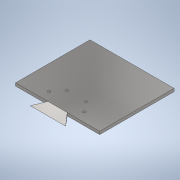
# Autodesk Inventor part: Part12
Saved by Autodesk Inventor 2022.3 (Build 263350000, 350)
## iProperties
Created: 2022-11-17
Part Number: Part12
Material: Steel, Alloy
Document SubType Name: Modeling
Designer: komputer
Density: 7.73 g/cm^3
Appearance: Semi-Polished
Mass: 236.899 g
Surface Area: 193.708 cm^2
Volume: 30.6467 cm^3
Author: komputer
Autodesk Inventor part; units mm, degrees
ref_plane "YZ Plane" through (0, 0, 0) normal (1, 0, 0) x (0, 1, 0)
ref_plane "XZ Plane" through (0, 0, 0) normal (0, 1, 0) x (-1, 0, 0)
ref_plane "XY Plane" through (0, 0, 0) normal (0, 0, 1) x (1, 0, 0)
sketch "Sketch1" plane through (0, 0, 0) normal (0, 1, 0) x (-1, 0, 0)
  line L0 (-8.4349, 11.6133) -> (91.5651, 11.6133)
  line L1 (91.5651, 11.6133) -> (91.5651, -88.3867)
  line L2 (91.5651, -88.3867) -> (-8.4349, -88.3867)
  line L3 (-8.4349, -88.3867) -> (-8.4349, 11.6133)
  point P0 (0, 0)
  dimension "d0" = 100
  dimension "d1" = 100
  constraints: 8 end point, 2 parallel, 1 horizontal, 1 perpendicular
  measures "d0" distance of L1.end L2.end
  measures "d1" distance of L0.end L1.end
extrude "Extrusion1" add sketch "Sketch1" along normal blind 3.5
sketch "Sketch2" plane through (-91.5651, 0, -88.3867) normal (-1, 0, 0) x (0, 0, 1)
  line L0 (0, 0) -> (100, 0) projected
  line L1 (100, 0) -> (100, 3.5) projected
  line L2 (0, 3.5) -> (100, 3.5) projected
  line L3 (0, 0) -> (0, 3.5) projected
  line L4 (0, 3.5) -> (100, 3.5) projected
  line L5 (100, 3.5) -> (90, 3.5)
  line L6 (0, 0) -> (100, 0) projected
  line L7 (90, 3.5) -> (100, 0)
  point P0 (88.3867, 0)
  dimension "d4" = 10
  constraints: 4 end point, 1 point on line
  measures "d4" distance of L1.end L5.end
extrude "Extrusion2" cut sketch "Sketch2" against normal through all contours L7 L2 L1
sketch "Sketch3" plane through (0, 3.5, 0) normal (0, 1, 0) x (1, 0, 0)
  line L0 (-91.5651, -1.6133) -> (8.4349, -1.6133) projected
  line L1 (8.4349, -1.6133) -> (8.4349, 88.3867) projected
  line L2 (8.4349, 88.3867) -> (-91.5651, 88.3867) projected
  line L3 (-91.5651, 88.3867) -> (-91.5651, -1.6133) projected
  line L4 (8.4349, -1.6133) -> (8.4349, -11.6133) projected
  line L5 (-91.5651, -1.6133) -> (8.4349, -1.6133) projected
  line L6 (-91.5651, -11.6133) -> (-91.5651, -1.6133) projected
  line L7 (-91.5651, -11.6133) -> (8.4349, -11.6133) projected
  line L8 (-91.5651, -11.6133) -> (8.4349, -11.6133) projected
  line L9 (8.4349, 88.3867) -> (-91.5651, 88.3867) projected
  line L10 (-91.5651, 88.3867) -> (-91.5651, -11.6133) projected
  line L11 (-41.5651, -11.6133) -> (8.4349, -11.6133)
  line L12 (-91.5651, -11.6133) -> (-41.5651, -11.6133)
  line L13 (-16.5651, -11.6133) -> (8.4349, -11.6133)
  line L14 (-91.5651, -11.6133) -> (-66.5651, -11.6133)
  line L15 (-16.5651, -11.6133) -> (-4.0651, -11.6133)
  line L16 (-79.0651, -11.6133) -> (-66.5651, -11.6133)
  line L17 (-41.5651, 25.8867) -> (-72.8151, -11.6133)
  line L18 (-41.5651, 25.8867) -> (-10.3151, -11.6133)
  line L19 (-28.2288, 9.8831) -> (-18.6484, -1.6133)
  line L20 (-91.5651, -1.6133) -> (8.4349, -1.6133) projected
  circle A0 centre (-30.1493, 12.1878) radius 1.6
  circle A1 centre (-20.569, 0.6914) radius 1.6
  line L21 (-18.6484, -1.6133) -> (-20.569, 0.6914)
  line L22 (-41.5651, 25.8867) -> (-41.5651, -11.6133)
  circle A2 centre (-52.9808, 12.1878) radius 1.6
  circle A3 centre (-62.5612, 0.6914) radius 1.6
  point P0 (0, 0)
  point P1 (-63.1373, 0)
  dimension "d15" = 3.2
  dimension "d16" = 3.2
  dimension "d17" = 3
  constraints: 22 end point, 7 midpoint, 6 point on line, 5 collinear, 4 centre point, 2 horizontal, 2 symmetric about line, 1 vertical, 2 other
  measures "d15" diameter of A0
  measures "d16" diameter of A1
  measures "d17" distance of L21.start L21.end
extrude "Extrusion3" cut sketch "Sketch3" against normal through all contours A1 L18 | L18 A1 | A3 L17 | L17 A3 | A2 L17 | L17 A2 | A0 L18 | L18 A0
sketch "Sketch4" plane through (0, 0, 0) normal (0, -1, 0) x (1, 0, 0)
  circle A0 centre (-52.9808, -12.1878) radius 1.6 projected
  circle A1 centre (-20.569, -0.6914) radius 1.6 projected
  circle A2 centre (-62.5612, -0.6914) radius 1.6 projected
  circle A3 centre (-30.1493, -12.1878) radius 1.6 projected
  line L0 (8.4349, -88.3867) -> (-91.5651, -88.3867) projected
  line L1 (8.4349, 11.6133) -> (8.4349, -88.3867) projected
  line L2 (-91.5651, 11.6133) -> (8.4349, 11.6133) projected
  line L3 (-91.5651, -88.3867) -> (-91.5651, 11.6133) projected
  line L4 (-91.5651, -88.3867) -> (-91.5651, 11.6133) projected
  line L5 (-91.5651, 11.6133) -> (8.4349, 11.6133)
  line L6 (8.4349, 11.6133) -> (8.4349, 21.6133)
  line L7 (8.4349, 21.6133) -> (-91.5651, 21.6133)
  line L8 (-91.5651, 21.6133) -> (-91.5651, 11.6133)
  line L9 (8.4349, 11.6133) -> (8.4349, -88.3867) projected
  line L10 (-91.5651, -88.3867) -> (8.4349, -88.3867)
  line L11 (8.4349, -88.3867) -> (8.4349, -78.3867)
  line L12 (8.4349, -78.3867) -> (-91.5651, -78.3867)
  line L13 (-91.5651, -78.3867) -> (-91.5651, -88.3867)
  line L14 (-91.5651, 1.6133) -> (8.4349, 1.6133) projected
  line L15 (-91.5651, 11.6133) -> (8.4349, 11.6133)
  line L16 (8.4349, 11.6133) -> (8.4349, 1.6133)
  line L17 (8.4349, 1.6133) -> (-91.5651, 1.6133)
  line L18 (-91.5651, 1.6133) -> (-91.5651, 11.6133)
  ellipse E0 centre (-76.8987, 15.9252) end of major axis (-87.6538, 6.9626) minor radius 2.0831 projected
  point P0 (0, 0)
  dimension "d20" = 10
  dimension "d21" = 10
  constraints: 24 end point, 6 parallel, 3 horizontal, 3 perpendicular, 1 point on line, 1 other
  measures "d20" distance of L6.end L5.end
  measures "d21" distance of L11.end L10.end
extrude "Extrusion4" add sketch "Sketch4" against normal up to surface (3.5 mm away) contours L14 L3 L2 E0 L1 | L2 E0 L7 L6 | L8 L7 E0 L2 | E0 L2 | L2 E0 L7
sketch "Sketch5" plane through (0, 0, 0) normal (0, -1, 0) x (1, 0, 0)
  line L0 (-91.5651, -88.3867) -> (-91.5651, 21.6133) projected
  line L1 (8.4349, -88.3867) -> (-91.5651, -88.3867) projected
  line L2 (8.4349, -88.3867) -> (8.4349, 21.6133) projected
  line L3 (8.4349, 21.6133) -> (-91.5651, 21.6133) projected
  circle A0 centre (-30.1493, -12.1878) radius 1.6 projected
  circle A1 centre (-62.5612, -0.6914) radius 1.6 projected
  circle A2 centre (-20.569, -0.6914) radius 1.6 projected
  circle A3 centre (-52.9808, -12.1878) radius 1.6 projected
  line L4 (-91.5651, -88.3867) -> (-91.5651, 21.6133) projected
  line L5 (8.4349, -88.3867) -> (-91.5651, -88.3867)
  line L6 (-91.5651, -88.3867) -> (-91.5651, -78.3867)
  line L7 (-91.5651, -78.3867) -> (8.4349, -78.3867)
  line L8 (8.4349, -78.3867) -> (8.4349, -88.3867)
  point P0 (0, 0)
  dimension "d24" = 10
  constraints: 8 end point, 2 parallel, 1 horizontal, 1 perpendicular, 1 point on line
  measures "d24" distance of L5.end L6.end
extrude "Extrusion5" cut sketch "Sketch5" against normal through all contours L0 L7 L2 L1
sketch "Sketch6" plane through (-91.5651, 0, 21.6133) normal (-1, 0, 0) x (0, 0, 1)
  line L0 (-100, 3.5) -> (-100, 0) projected
  line L1 (-100, 0) -> (0, 0) projected
  line L2 (0, 0) -> (0, 3.5) projected
  line L3 (0, 3.5) -> (-100, 3.5) projected
  line L4 (-6.5312, 3.5) -> (-20.2018, 3.5) projected
  line L5 (-6.5312, 8.5) -> (-6.5312, 3.5) projected
  line L6 (-20.2018, 8.5) -> (-6.5312, 8.5) projected
  line L7 (-20.2018, 3.5) -> (-20.2018, 8.5) projected
  line L8 (-100, 0) -> (0, 0) projected
  line L9 (0, 0) -> (-11.4782, 3.5)
  line L10 (0, 3.5) -> (-100, 3.5) projected
  point P0 (-21.6133, 0)
  dimension "d27" = 12
  constraints: 2 end point, 1 point on line
  measures "d27" distance of L1.end L9.end
extrude "Extrusion6" cut sketch "Sketch6" against normal through all contours L9 L3 L2
sketch "Sketch7" plane through (0, 3.5, 0) normal (0, 1, 0) x (1, 0, 0)
  line L0 (-91.5651, -10.1351) -> (8.4349, -10.1351) projected
  line L1 (8.4349, -10.1351) -> (8.4349, 78.3867) projected
  line L2 (8.4349, 78.3867) -> (-91.5651, 78.3867) projected
  line L3 (-91.5651, -10.1351) -> (-91.5651, 78.3867) projected
  circle A0 centre (-52.9808, 12.1878) radius 1.6 projected
  circle A1 centre (-20.569, 0.6914) radius 1.6 projected
  circle A2 centre (-62.5612, 0.6914) radius 1.6 projected
  circle A3 centre (-30.1493, 12.1878) radius 1.6 projected
  line L4 (8.4349, -10.1351) -> (8.4349, -21.6133) projected
  line L5 (-91.5651, -10.1351) -> (8.4349, -10.1351) projected
  line L6 (-91.5651, -21.6133) -> (-91.5651, -10.1351) projected
  line L7 (8.4349, -21.6133) -> (-91.5651, -21.6133) projected
  circle A4 centre (-30.1493, 12.1878) radius 1.6 projected
  circle A5 centre (-20.569, 0.6914) radius 1.6 projected
  line L8 (-30.1493, 12.1878) -> (-20.569, 0.6914)
  line L9 (-91.5651, -10.1351) -> (8.4349, -10.1351) projected
  line L10 (-30.1493, -10.1351) -> (-20.569, -21.6133)
  line L11 (8.4349, -21.6133) -> (-91.5651, -21.6133) projected
  circle A6 centre (-62.5612, 0.6914) radius 1.6 projected
  line L12 (-52.9808, 12.1878) -> (-62.5612, 0.6914)
  line L13 (-52.9808, -10.1351) -> (-62.5612, -21.6133)
  point P0 (0, 0)
  constraints: 8 end point, 4 point on line
extrude "Extrusion7" cut sketch "Sketch7" against normal blind 10 contours L0 L13 L7 L6 | L0 L4 L7 L10
sketch "Sketch8" plane through (0, 3.5, 0) normal (0, 1, 0) x (1, 0, 0)
  line L0 (-91.5651, -10.1351) -> (-52.9808, -10.1351) projected
  line L1 (-52.9808, -10.1351) -> (-30.1493, -10.1351) projected
  line L2 (-30.1493, -10.1351) -> (8.4349, -10.1351) projected
  line L3 (8.4349, -10.1351) -> (8.4349, 78.3867) projected
  line L4 (8.4349, 78.3867) -> (-91.5651, 78.3867) projected
  line L5 (-91.5651, -10.1351) -> (-91.5651, 78.3867) projected
  circle A0 centre (-52.9808, 12.1878) radius 1.6 projected
  circle A1 centre (-20.569, 0.6914) radius 1.6 projected
  circle A2 centre (-62.5612, 0.6914) radius 1.6 projected
  circle A3 centre (-30.1493, 12.1878) radius 1.6 projected
  line L6 (8.4349, -10.1351) -> (8.4349, 78.3867) projected
  line L7 (8.4349, -10.1351) -> (-30.1493, -10.1351)
  line L8 (-30.1493, -10.1351) -> (-30.1493, -7.1351)
  line L9 (-30.1493, -7.1351) -> (8.4349, -7.1351)
  line L10 (8.4349, -7.1351) -> (8.4349, -10.1351)
  line L11 (-91.5651, -10.1351) -> (-52.9808, -10.1351)
  line L12 (-52.9808, -10.1351) -> (-52.9808, -7.1351)
  line L13 (-52.9808, -7.1351) -> (-91.5651, -7.1351)
  line L14 (-91.5651, -7.1351) -> (-91.5651, -10.1351)
  point P0 (0, 0)
  dimension "d32" = 3
  constraints: 16 end point, 4 parallel, 2 horizontal, 2 perpendicular, 1 point on line
  measures "d32" distance of L7.end L8.end
extrude "Extrusion8" cut sketch "Sketch8" against normal through all contours L5 L13 L12 L0 | L8 L9 L3 L2
sketch "Sketch9" plane through (0, 3.5, 0) normal (0, 1, 0) x (1, 0, 0)
  circle A0 centre (-30.1493, 12.1878) radius 1.6 projected
  circle A1 centre (-62.5612, 0.6914) radius 1.6 projected
  circle A2 centre (-20.569, 0.6914) radius 1.6 projected
  circle A3 centre (-52.9808, 12.1878) radius 1.6 projected
  line L0 (-91.5651, -7.1351) -> (-52.9808, -7.1351) projected
  line L1 (-52.9808, -7.1351) -> (-52.9808, -10.1351) projected
  line L2 (-52.9808, -10.1351) -> (-30.1493, -10.1351) projected
  line L3 (-30.1493, -10.1351) -> (-30.1493, -7.1351) projected
  line L4 (-30.1493, -7.1351) -> (8.4349, -7.1351) projected
  line L5 (8.4349, -7.1351) -> (8.4349, 78.3867) projected
  line L6 (8.4349, 78.3867) -> (-91.5651, 78.3867) projected
  line L7 (-91.5651, -7.1351) -> (-91.5651, 78.3867) projected
  line L8 (-91.5651, 78.3867) -> (-91.5651, -7.1351) projected
  line L9 (8.4349, 78.3867) -> (8.4349, -7.1351) projected
  line L10 (-91.5651, 78.3867) -> (8.4349, 78.3867)
  line L11 (8.4349, 78.3867) -> (8.4349, 73.3867)
  line L12 (8.4349, 73.3867) -> (-91.5651, 73.3867)
  line L13 (-91.5651, 73.3867) -> (-91.5651, 78.3867)
  line L14 (-91.5651, 78.3867) -> (8.4349, 78.3867) projected
  line L15 (-41.5651, 78.3867) -> (-41.5651, 59.9995)
  line L16 (-41.5651, 59.9995) -> (-16.5651, 59.9995)
  line L17 (-16.5651, 59.9995) -> (-66.5651, 59.9995)
  line L18 (8.4349, 73.3867) -> (-16.5651, 73.3867)
  line L19 (-16.5651, 73.3867) -> (-16.5651, 45.3867)
  line L20 (-16.5651, 45.3867) -> (8.4349, 45.3867)
  line L21 (8.4349, 45.3867) -> (8.4349, 73.3867)
  line L22 (-66.5651, 73.3867) -> (-79.5403, 73.3867)
  line L23 (-79.5403, 73.3867) -> (-79.5403, 45.3867)
  line L24 (-79.5403, 45.3867) -> (-66.5651, 45.3867)
  line L25 (-66.5651, 45.3867) -> (-66.5651, 73.3867)
  line L26 (-91.5651, 45.3867) -> (-66.5651, 45.3867)
  line L27 (-66.5651, 45.3867) -> (-66.5651, 78.3867)
  line L28 (-66.5651, 78.3867) -> (-91.5651, 78.3867)
  line L29 (-91.5651, 78.3867) -> (-91.5651, 45.3867)
  line L30 (-14.4969, 45.3867) -> (-14.4969, 50.3867)
  line L31 (-14.4969, 50.3867) -> (-14.4969, 78.3867)
  line L32 (-14.4969, 64.3867) -> (-82.4701, 64.3867)
  line L33 (-82.4701, 64.3867) -> (-3.1512, 64.3867)
  line L34 (-14.4969, 64.3867) -> (-9.1279, 64.3867)
  line L35 (-9.1279, 64.3867) -> (-9.1279, 62.3867)
  line L36 (-9.1279, 62.3867) -> (-14.4969, 62.3867)
  line L37 (-14.4969, 62.3867) -> (-14.4969, 64.3867)
  line L38 (-14.4969, 64.3867) -> (-9.1279, 64.3867)
  line L39 (-9.1279, 64.3867) -> (-9.1279, 66.3867)
  line L40 (-9.1279, 66.3867) -> (-14.4969, 66.3867)
  line L41 (-14.4969, 66.3867) -> (-14.4969, 64.3867)
  line L42 (-66.5651, 64.3867) -> (-72.2729, 64.3867)
  line L43 (-72.2729, 64.3867) -> (-72.2729, 62.3867)
  line L44 (-72.2729, 62.3867) -> (-66.5651, 62.3867)
  line L45 (-66.5651, 62.3867) -> (-66.5651, 64.3867)
  line L46 (-72.2729, 62.3867) -> (-66.5651, 62.3867)
  line L47 (-66.5651, 62.3867) -> (-66.5651, 66.3867)
  line L48 (-66.5651, 66.3867) -> (-72.2729, 66.3867)
  line L49 (-72.2729, 66.3867) -> (-72.2729, 62.3867)
  line L50 (-14.4969, 73.3867) -> (-14.4969, 66.3867)
  line L51 (-9.1279, 66.3867) -> (-14.4969, 66.3867)
  line L52 (-9.1279, 66.3867) -> (-9.1279, 62.3867)
  line L53 (-14.4969, 62.3867) -> (-14.4969, 45.3867)
  line L54 (-14.4969, 62.3867) -> (-9.1279, 62.3867)
  line L55 (-14.4969, 45.3867) -> (8.4349, 45.3867)
  line L56 (-14.4969, 66.3867) -> (-16.5651, 66.3867)
  line L57 (-14.4969, 62.3867) -> (-16.5651, 62.3867)
  point P0 (0, 0)
  dimension "d35" = 5
  dimension "d36" = 25
  dimension "d37" = 50
  dimension "d38" = 28
  dimension "d39" = 28
  dimension "d40" = 5
  dimension "d41" = 2
  dimension "d42" = 2
  constraints: 94 end point, 19 point on line, 17 parallel, 10 horizontal, 10 perpendicular, 5 collinear, 2 midpoint, 2 vertical
  measures "d35" distance of L10.end L11.end
  measures "d36" distance of L15.end L16.end
  measures "d37" distance of L16.end L17.end
  measures "d38" distance of L19.end L18.end
  measures "d39" distance of L23.end L22.end
  measures "d40" distance of L30.start L30.end
  measures "d41" distance of L34.end L35.end
  measures "d42" distance of L39.end L38.end
extrude "Extrusion9" cut sketch "Sketch9" against normal through all contours L7 L12 L23 L26 | L7 L6 L27 L12 | L23 L32 L43 L44 L25 L24 | L12 L25 L48 L49 L32 L23 | L6 L15 L12 L27 | L6 L31 L12 L15 | L20 L30 L31 L36 L35 L39 L40 L12 L5 | L6 L5 L12 L31 | L12 L31 L56 L19 | L19 L57 L31 L30 L20
body "Solid1"
